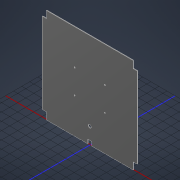
# Autodesk Inventor part: Panel Bottom
Saved by Autodesk Inventor 2022.2 (Build 262287010, 287A)
## iProperties
Created: 2022-03-16
Part Number: Panel Bottom
Material: Polycarbonat, klar
Document SubType Name: Modeling
Designer: sleib
Density: 1.2 g/cm^3
Appearance: Glatt - Schwarz
Author: sleib
Autodesk Inventor part; units mm, degrees
ref_plane "YZ Plane" through (0, 0, 0) normal (1, 0, 0) x (0, 1, 0)
ref_plane "XZ Plane" through (0, 0, 0) normal (0, 1, 0) x (-1, 0, 0)
ref_plane "XY Plane" through (0, 0, 0) normal (0, 0, 1) x (1, 0, 0)
sketch "Skizze1" plane through (0, 0, 0) normal (0, 0, 1) x (1, 0, 0)
  line L0 (-235, -235) -> (235, -235)
  line L1 (235, -235) -> (235, 235)
  line L2 (235, 235) -> (-235, 235)
  line L3 (-235, 235) -> (-235, -235)
  line L4 (-235, -235) -> (235, 235) construction
  line L5 (235, -235) -> (-235, 235) construction
  line L6 (-235, -235) -> (-215, -235)
  line L7 (-215, -235) -> (-215, -200)
  line L8 (-215, -200) -> (-235, -200)
  line L9 (-235, -200) -> (-235, -235)
  line L10 (235, -235) -> (215, -235)
  line L11 (215, -235) -> (215, -200)
  line L12 (215, -200) -> (235, -200)
  line L13 (235, -200) -> (235, -235)
  line L14 (235, 235) -> (215, 235)
  line L15 (215, 235) -> (215, 200)
  line L16 (215, 200) -> (235, 200)
  line L17 (235, 200) -> (235, 235)
  line L18 (-235, 235) -> (-215, 235)
  line L19 (-215, 235) -> (-215, 200)
  line L20 (-215, 200) -> (-235, 200)
  line L21 (-235, 200) -> (-235, 235)
  line L22 (-10, -235) -> (10, -235)
  line L23 (10, -235) -> (10, -215)
  line L24 (10, -215) -> (-10, -215)
  line L25 (-10, -215) -> (-10, -235)
  circle A0 centre (0, -155) radius 7.5
  circle A1 centre (-75, 60) radius 3
  circle A2 centre (75, 60) radius 3
  circle A3 centre (75, -60) radius 3
  circle A4 centre (-75, -60) radius 3
  line L26 (-75, -60) -> (75, -60) construction
  line L27 (75, -60) -> (75, 60) construction
  line L28 (75, 60) -> (-75, 60) construction
  line L29 (-75, 60) -> (-75, -60) construction
  line L30 (-75, -60) -> (75, 60) construction
  line L31 (75, -60) -> (-75, 60) construction
  point P0 (0, 0)
  point P1 (0, -235)
  dimension "d0" = 470
  dimension "d1" = 470
  dimension "d4" = 35
  dimension "d5" = 20
  dimension "d6" = 20
  dimension "d7" = 20
  dimension "d8" = 15
  dimension "d9" = 80
  dimension "d10" = 150
  dimension "d11" = 120
  dimension "d12" = 6
  constraints: 64 end point, 14 parallel, 7 horizontal, 7 perpendicular, 6 equal length, 6 midpoint, 5 centre point, 3 coincident, 3 equal radius, 1 point on line, 1 vertical alignment
  measures "d0" distance of L2.end L1.end
  measures "d1" distance of L1.end L0.end
  measures "d4" distance of L18.end L19.end
  measures "d5" distance of L19.end L20.end
  measures "d6" distance of L23.end L24.end
  measures "d7" distance of L24.end L22.start
  measures "d8" diameter of A0
  measures "d9" distance from line of L0 A0.centre
  measures "d10" distance of L27.end L28.end
  measures "d11" distance of L26.end L27.end
  measures "d12" diameter of A1
extrude "Extrusion1" add sketch "Skizze1" along normal blind 3 contours L7 L8 L3 L20 L19 L2 L15 L16 L1 L12 L11 L0 L23 L24 L25
